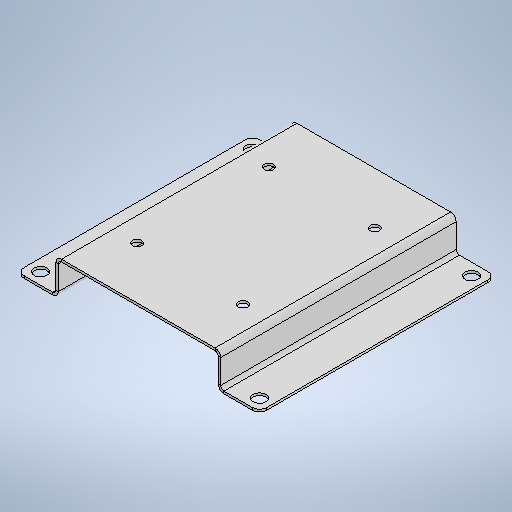
# Autodesk Inventor part: TKS mixer support
Saved by Autodesk Inventor 2025.3 (Build 293356030, 356C)
## iProperties
Created: 2025-08-15
Part Number: TKS mixer support
Material: Stainless Steel
Document SubType Name: Sheet Metal
Designer: admin
Mass: 1762.25 g
Surface Area: 2283.33 cm^2
Volume: 220.281 cm^3
Density: 8 g/cm^3
Sheet Metal Rule: AISI304 2mm Die16
Sheet Metal Width: 200,000 mm
Sheet Metal Length: 254,808 mm
Sheet Metal Area: 50961,593 mm^2
Appearance: Default
Flat Pattern Width: 20 cm
Flat Pattern Length: 25.4808 cm
Flat Pattern Area: 509.616 cm^2
Author: admin
Autodesk Inventor part; units mm, degrees
ref_plane "YZ Plane" through (0, 0, 0) normal (1, 0, 0) x (0, 1, 0)
ref_plane "XZ Plane" through (0, 0, 0) normal (0, 1, 0) x (-1, 0, 0)
ref_plane "XY Plane" through (0, 0, 0) normal (0, 0, 1) x (1, 0, 0)
sketch "Sketch1" plane through (0, 0, 0) normal (0, 0, 1) x (1, 0, 0)
  line L0 (-70, -100) -> (70, -100)
  line L1 (70, -100) -> (70, 100)
  line L2 (70, 100) -> (-70, 100)
  line L3 (-70, 100) -> (-70, -100)
  line L4 (-70, -100) -> (70, 100) construction
  line L5 (70, -100) -> (-70, 100) construction
  point P0 (0, 0)
  dimension "d154" = 140
  dimension "d155" = 200
  measures "d154" distance of L1.end L2.end
  measures "d155" distance of L0.end L1.end
extrude "Plate5" add sketch "Sketch1" along normal blind 2
sketch "Sketch7" plane through (68, -100, 2) normal (1, 0, 0) x (0, 1, 0)
  line L0 (200, 0) -> (0, 0)
  line L1 (0, 0) -> (0, -30)
  line L2 (0, -30) -> (200, -30)
  line L3 (200, -30) -> (200, 0)
  constraints: 6 end point, 1 horizontal, 1 perpendicular, 1 vertical
edge flange "Flange3" height 30 angle 90 thickness 2 bend radius 2.75 thickness toward (1, 0, 0) relief round relief width 2 relief depth 1 corner gap 2.75 corner form 0 edges at (70, 0, 0) (-70, 0, 0) wall of the first edge with corners at (68, 100, 2) (68, -100, 2) (68, -100, -28) (68, 100, -28)
bend "Bend3"
corner "Corner3"
sketch "Sketch8" plane through (-68, -100, -26) normal (0, 0, -1) x (-1, 0, 0)
  line L0 (0, 200) -> (0, 0)
  line L1 (0, 0) -> (35, 0)
  line L2 (35, 0) -> (35, 200)
  line L3 (35, 200) -> (0, 200)
  constraints: 6 end point, 1 horizontal, 1 perpendicular, 1 vertical
edge flange "Flange4" height 35 angle 90 thickness 2 bend radius 2.75 thickness toward (0, 0, -1) relief round relief width 2 relief depth 1 corner gap 2.75 corner form 0 edges at (-70, 0, -28) (70, 0, -28) wall of the first edge with corners at (-68, 100, -26) (-68, -100, -26) (-103, -100, -26) (-103, 100, -26)
bend "Bend4"
corner "Corner4"
sketch "Sketch9" plane through (-103, -100, -26) normal (0, 0, 1) x (1, 0, 0)
  line L0 (30.25, 0) -> (30.25, 200) projected
  line L1 (30.25, 200) -> (0, 200) projected
  line L2 (0, 200) -> (0, 0) projected
  line L3 (30.25, 0) -> (0, 0) projected
  circle A0 centre (10, 190) radius 5.5
  circle A1 centre (10, 10) radius 5.5
  point P0 (103, 100)
  dimension "d177" = 11
  dimension "d178" = 10
  dimension "d179" = 10
  dimension "d180" = 10
  constraints: 2 centre point, 1 equal radius, 1 vertical alignment
  measures "d177" diameter of A0
  measures "d178" distance from line of A0.centre L1
  measures "d179" distance from line of L2 A0.centre
  measures "d180" distance from line of L3 A1.centre
extrude "Cut1" cut sketch "Sketch9" against normal blind 2 contours A0 | A1
mirror "Mirror1" about plane through (0, 0, 0) normal (1, 0, 0) of "Cut1"
fillet "Corner Round2" radius 6 4 edges at (-103, 100, -27) (-103, -100, -27) (103, 100, -27) (103, -100, -27)
sketch "Sketch10" plane through (0, 0, 2) normal (0, 0, 1) x (1, 0, 0)
  circle A0 centre (-45, 56) radius 4
  line L0 (-45, 56) -> (45, 56) construction
  line L1 (45, 56) -> (45, -56) construction
  line L2 (45, -56) -> (-45, -56) construction
  line L3 (-45, -56) -> (-45, 56) construction
  circle A1 centre (45, 56) radius 4
  circle A2 centre (45, -56) radius 4
  circle A3 centre (-45, -56) radius 4
  point P0 (0, 0)
  point P1 (0, 56)
  point P2 (45, 0)
  dimension "d185" = 8
  dimension "d186" = 90
  dimension "d187" = 112
  constraints: 8 end point, 4 centre point, 3 coincident, 3 equal radius, 2 midpoint, 2 parallel, 1 horizontal, 1 horizontal alignment, 1 perpendicular, 1 vertical alignment
  measures "d185" diameter of A0
  measures "d186" distance of L0.start L1.start
  measures "d187" distance of L1.start L1.end
extrude "Cut2" cut sketch "Sketch10" against normal blind 2
body "Solid3"
